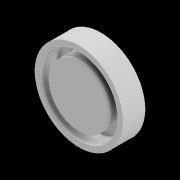
# Autodesk Inventor part: 螺旋鉤子底座
Saved by Autodesk Inventor 2020 (Build 240168000, 168)
## iProperties
Created: 2021-04-09
Part Number: 螺旋鉤子底座
Material: 一般
Document SubType Name: Modeling
Designer: 88690
Density: 1 g/cm^3
Appearance: 預設
Author: 88690
Autodesk Inventor part; units mm, degrees
ref_plane "YZ Plane" through (0, 0, 0) normal (1, 0, 0) x (0, 1, 0)
ref_plane "XZ Plane" through (0, 0, 0) normal (0, 1, 0) x (-1, 0, 0)
ref_plane "XY Plane" through (0, 0, 0) normal (0, 0, 1) x (1, 0, 0)
sketch "草圖1" plane through (0, 0, 0) normal (0, 0, 1) x (1, 0, 0)
  circle A0 centre (0, 0) radius 80
  circle A1 centre (0, 0) radius 70
  circle A2 centre (0, 0) radius 55
  dimension "d0" = 160
  dimension "d1" = 140
  dimension "d2" = 110
  constraints: 3 centre point, 3 coincident
  measures "d0" diameter of A0
  measures "d1" diameter of A1
  measures "d2" diameter of A2
extrude "擠出1" add sketch "草圖1" against normal blind 30
sketch "草圖2" plane through (0, 0, -30) normal (0, 0, -1) x (-1, 0, 0)
  circle A0 centre (0, 0) radius 80 projected
extrude "擠出2" add sketch "草圖2" along normal blind 10
sketch "草圖3" plane through (0, 0, -40) normal (0, 0, -1) x (-1, 0, 0)
  circle A0 centre (0, 0) radius 25
  dimension "d7" = 50
  constraints: 1 centre point, 1 coincident
  measures "d7" diameter of A0
sketch "草圖4" plane through (0, 0, 0) normal (0, 0, 1) x (1, 0, 0)
  circle A0 centre (0, 0) radius 80 projected
  circle A1 centre (0, 0) radius 70 projected
  line L0 (0, 0) -> (-69.282, -40) construction
  line L1 (0, 0) -> (69.282, -40) construction
  line L2 (0, 0) -> (80, 0) construction
  line L3 (0, 0) -> (-80, 0) construction
  circle A2 centre (0, 0) radius 80 projected
  line L4 (-69.282, -40) -> (-61.4878, -35.5)
  line L5 (69.282, -40) -> (61.4878, -35.5)
  circle A3 centre (0, 0) radius 70 projected
  arc A4 (-61.4878, -35.5) -> (61.4878, -35.5) centre (0, 0) ccw
  dimension "d10" = 30
  dimension "d11" = 30
  dimension "d13" = 71
  constraints: 12 end point, 6 point on circle, 2 collinear, 2 horizontal, 1 centre point, 3 other
  measures "d10" angle of L3 L0
  measures "d11" angle of L2 L1
  measures "d13" radius of A4
sketch "草圖5" plane through (0, 0, 0) normal (0, 1, 0) x (-1, 0, 0)
  line L0 (-59.2626, 395) -> (59.2626, 395) construction
  line L1 (0, 0) -> (0, 395) construction
  line L2 (66.7748, 395) -> (-66.7748, 395) construction
  line L3 (67.5187, 0) -> (67.5187, 395) construction
  line L4 (-67.5187, 0) -> (-67.5187, 395) construction
  arc A0 (67.5187, 375.1961) -> (-67.5187, 375.1961) centre (0, 270) ccw
  line L5 (67.5187, 375.1961) -> (67.5187, 415)
  line L6 (-67.5187, 375.1961) -> (-67.5187, 415)
  line L7 (-67.5187, 415) -> (67.5187, 415)
  dimension "d19" = 125
  dimension "d20" = 20
  constraints: 8 end point, 3 point on line, 2 point on circle, 2 vertical, 1 centre point, 1 horizontal, 1 midpoint, 1 tangent
  measures "d19" radius of A0
  measures "d20" distance between parallel lines of L0 L7
